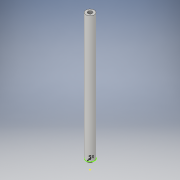
# Autodesk Inventor part: Stangen
Saved by Autodesk Inventor 2019.5 (Build 235369000, 369)
## iProperties
Created: 2021-09-30
Part Number: Stangen
Material: Generisch
Document SubType Name: Modeling
Designer: mritt
Density: 1 g/cm^3
Appearance: Vorgabe
Author: mritt
Autodesk Inventor part; units mm, degrees
ref_plane "YZ Plane" through (0, 0, 0) normal (1, 0, 0) x (0, 1, 0)
ref_plane "XZ Plane" through (0, 0, 0) normal (0, 1, 0) x (-1, 0, 0)
ref_plane "XY Plane" through (0, 0, 0) normal (0, 0, 1) x (1, 0, 0)
sketch "Skizze1" plane through (0, 0, 0) normal (0, 1, 0) x (-1, 0, 0)
  circle A0 centre (11.4284, -11.664) radius 5
  circle A1 centre (11.4284, -11.664) radius 2.5
  point P0 (0, 0)
  dimension "d0" = 10
  dimension "d1" = 5
  constraints: 2 centre point, 1 coincident
  measures "d0" diameter of A0
  measures "d1" diameter of A1
extrude "Extrusion1" add sketch "Skizze1" along normal blind 150 contours A0 | A1
extrude "Extrusion2" add sketch "Skizze1" against normal blind 3 contours A1
thread "Gewinde1" size "M5x0.8" class "6g" standard "ANSI Metric M Profile" full length
sketch "Skizze2" plane through (-11.4284, 150, -11.664) normal (0, 1, 0) x (1, 0, 0)
  point P0 (11.4284, -11.664)
  point P1 (0, 0)
hole "Bohrung1" at (-11.4284, 150, -11.664) direction (0, -1, 0) diameter 4.978 depth 19.05 tip angle 118 thread size "1/4-20 UNC" class "2B" standard "ANSI Unified Screw Threads"
